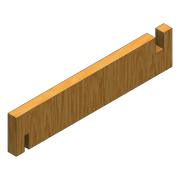
# Autodesk Inventor part: Sensor Holder
Saved by Autodesk Inventor 2016 (Build 200138000, 138)
## iProperties
Created: 2015-07-07
Part Number: Sensor Holder
Material: Plywood, Finish
Document SubType Name: Modeling
Designer: Sebastian
Density: 0.552 g/cm^3
Appearance: Plywood - New
Mass: 0.8901 g
Surface Area: 15.31 cm^2
Volume: 1.6125 cm^3
Author: Sebastian
Autodesk Inventor part; units mm, degrees
ref_plane "YZ Plane" through (0, 0, 0) normal (1, 0, 0) x (0, 1, 0)
ref_plane "XZ Plane" through (0, 0, 0) normal (0, 1, 0) x (-1, 0, 0)
ref_plane "XY Plane" through (0, 0, 0) normal (0, 0, 1) x (1, 0, 0)
sketch "Sketch1" plane through (0, 0, 0) normal (1, 0, 0) x (0, 1, 0)
  line L0 (56, 0) -> (56, -12)
  line L1 (0, -12) -> (0, 0)
  line L2 (50, 0) -> (50, -5)
  line L3 (50, -5) -> (53, -5)
  line L4 (53, -5) -> (53, 0)
  line L5 (56, 0) -> (53, 0)
  line L6 (50, 0) -> (0, 0)
  line L7 (4.5, -12) -> (4.5, -7)
  line L8 (4.5, -7) -> (3, -7)
  line L9 (3, -7) -> (3, -12)
  line L10 (56, -12) -> (4.5, -12)
  line L11 (3, -12) -> (0, -12)
  dimension "d0" = 56
  dimension "d4" = 3
  dimension "d5" = 5
  dimension "d6" = 3
  dimension "d8" = 5
  dimension "d9" = 3
  dimension "d11" = 12
  dimension "d12" = 0
  dimension "d13" = 0
  constraints: 24 end point, 3 parallel, 2 collinear
  measures "d0" distance of L0.end L1.start
  measures "d4" distance of L3.end L2.end
  measures "d5" distance of L2.end L2.start
  measures "d6" distance between parallel lines of L4 L0
  measures "d8" distance of L7.end L7.start
  measures "d9" distance between parallel lines of L1 L9
  measures "d11" distance between parallel lines of L10 L6
  measures "d12" distance between parallel lines of L10 L11
  measures "d13" distance between parallel lines of L6 L5
extrude "Extrusion1" add sketch "Sketch1" along normal blind 3
body "Solid1"
